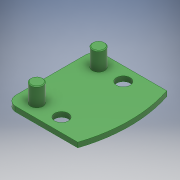
# Autodesk Inventor part: green_part-july21
Saved by Autodesk Inventor 2017 SP1 (Build 210196100, 196)
## iProperties
Created: 2016-07-25
Part Number: green_part-july21
Material: Plastique ABS
Document SubType Name: Modeling
Designer: tmonglon
Density: 1.06 g/cm^3
Appearance: Lisse - Vert forêt foncé
Author: tmonglon
Autodesk Inventor part; units mm, degrees
ref_plane "YZ Plane" through (0, 0, 0) normal (1, 0, 0) x (0, 1, 0)
ref_plane "XZ Plane" through (0, 0, 0) normal (0, 1, 0) x (-1, 0, 0)
ref_plane "XY Plane" through (0, 0, 0) normal (0, 0, 1) x (1, 0, 0)
sketch "Esquisse1" plane through (0, 0, 0) normal (0, 0, 1) x (1, 0, 0)
  line L0 (0, 0) -> (-29, 0)
  line L1 (-29, 0) -> (-29, 36)
  line L2 (-29, 36) -> (0, 36)
  line L3 (-24.5656, 33) -> (-19.5656, 33)
  line L4 (-19.5656, 33) -> (-19.5656, 28)
  line L5 (-19.5656, 28) -> (-24.5656, 28)
  line L6 (-24.5656, 28) -> (-24.5656, 33)
  line L7 (-14.5656, 33) -> (-9.5656, 33)
  line L8 (-9.5656, 33) -> (-9.5656, 28)
  line L9 (-9.5656, 28) -> (-14.5656, 28)
  line L10 (-14.5656, 28) -> (-14.5656, 33)
  line L11 (-24.5656, 8) -> (-19.5656, 8)
  line L12 (-19.5656, 8) -> (-19.5656, 3)
  line L13 (-19.5656, 3) -> (-24.5656, 3)
  line L14 (-24.5656, 3) -> (-24.5656, 8)
  line L15 (-14.5656, 8) -> (-9.5656, 8)
  line L16 (-9.5656, 8) -> (-9.5656, 3)
  line L17 (-9.5656, 3) -> (-14.5656, 3)
  line L18 (-14.5656, 3) -> (-14.5656, 8)
  arc A0 (0, 0) -> (0, 36) centre (-54.0833, 18) ccw
  line L19 (-9.3156, 33.25) -> (-14.8156, 33.25)
  line L20 (-14.8156, 33.25) -> (-14.8156, 27.75)
  line L21 (-14.8156, 27.75) -> (-9.3156, 27.75)
  line L22 (-9.3156, 27.75) -> (-9.3156, 33.25)
  line L23 (-9.3156, 8.25) -> (-14.8156, 8.25)
  line L24 (-14.8156, 8.25) -> (-14.8156, 2.75)
  line L25 (-14.8156, 2.75) -> (-9.3156, 2.75)
  line L26 (-9.3156, 2.75) -> (-9.3156, 8.25)
  dimension "d0" = 36
  dimension "d1" = 29
  dimension "d2" = 5
  dimension "d3" = 5
  dimension "d4" = 5
  dimension "d5" = 5
  dimension "d6" = 20
  dimension "d7" = 5
  dimension "d8" = 3
  dimension "d9" = 57
  dimension "d21" = 5.5
  dimension "d22" = 5.5
  constraints: 54 end point, 13 parallel, 8 point on line, 7 perpendicular, 5 horizontal, 2 point on circle, 1 centre point, 6 other
  measures "d0" distance of L0.end L1.end
  measures "d1" distance of L1.end L2.end
  measures "d2" distance of L5.end L3.start
  measures "d3" distance of L3.start L3.end
  measures "d4" distance of L7.start L7.end
  measures "d5" distance between parallel lines of L10 L4
  measures "d6" distance between parallel lines of L15 L9
  measures "d7" distance of L15.end L16.end
  measures "d8" distance between parallel lines of L0 L17
  measures "d9" radius of A0
  measures "d21" distance of L23.start L23.end
  measures "d22" distance of L20.end L21.end
extrude "Extrusion1" add sketch "Esquisse1" along normal blind 2 contours L0 L1 L2 A0 | L22 L21 L20 L19 | L26 L25 L24 L23
extrude "Extrusion3" add sketch "Esquisse1" along normal blind 9.5 contours L3 L4 L5 L6 | L11 L12 L13 L14
fillet "Congé1" radius 4 2 edges at (-29, 0, 1) (-29, 36, 1)
sketch "Esquisse2" plane through (0, 0, 2) normal (0, 0, 1) x (1, 0, 0)
  line L0 (-9.5656, 8) -> (-9.5656, 3) projected
  line L1 (-9.5656, 3) -> (-14.5656, 3) projected
  line L2 (-14.5656, 3) -> (-14.5656, 8) projected
  line L3 (-14.5656, 8) -> (-9.5656, 8) projected
  line L4 (-19.5656, 8) -> (-19.5656, 3) projected
  line L5 (-19.5656, 3) -> (-24.5656, 3) projected
  line L6 (-24.5656, 3) -> (-24.5656, 8) projected
  line L7 (-24.5656, 8) -> (-19.5656, 8) projected
  line L8 (-9.5656, 33) -> (-9.5656, 28) projected
  line L9 (-9.5656, 28) -> (-14.5656, 28) projected
  line L10 (-14.5656, 28) -> (-14.5656, 33) projected
  line L11 (-14.5656, 33) -> (-9.5656, 33) projected
  line L12 (-19.5656, 33) -> (-19.5656, 28) projected
  line L13 (-19.5656, 28) -> (-24.5656, 28) projected
  line L14 (-24.5656, 28) -> (-24.5656, 33) projected
  line L15 (-24.5656, 33) -> (-19.5656, 33) projected
  arc A0 (-25, 36) -> (-29, 32) centre (-25, 32) ccw projected
  line L16 (-29, 32) -> (-29, 4) projected
  arc A1 (-29, 4) -> (-25, 0) centre (-25, 4) ccw projected
  line L17 (-25, 0) -> (0, 0) projected
  arc A2 (0, 0) -> (0, 36) centre (-54.0833, 18) ccw projected
  line L18 (0, 36) -> (-25, 36) projected
  circle A3 centre (-12.0656, 30.5) radius 2.5
  circle A4 centre (-12.0656, 5.5) radius 2.5
  constraints: 6 tangent, 2 centre point
extrude "Extrusion4" add sketch "Esquisse2" against normal up to surface (2 mm away) contours L0 A4 L3 | L0 L1 A4 | A4 L2 L3 | L1 L2 A4 | L8 A3 L11 | L8 L9 A3 | A3 L10 L11 | L9 L10 A3
sketch "Esquisse3" plane through (0, 0, 9.5) normal (0, 0, 1) x (1, 0, 0)
  circle A0 centre (-12.0656, 5.5) radius 2.5 projected
  line L0 (-19.5656, 8) -> (-19.5656, 3) projected
  line L1 (-19.5656, 3) -> (-24.5656, 3) projected
  line L2 (-24.5656, 3) -> (-24.5656, 8) projected
  line L3 (-24.5656, 8) -> (-19.5656, 8) projected
  circle A1 centre (-12.0656, 30.5) radius 2.5 projected
  line L4 (-19.5656, 33) -> (-19.5656, 28) projected
  line L5 (-19.5656, 28) -> (-24.5656, 28) projected
  line L6 (-24.5656, 28) -> (-24.5656, 33) projected
  line L7 (-24.5656, 33) -> (-19.5656, 33) projected
  arc A2 (-25, 36) -> (-29, 32) centre (-25, 32) ccw projected
  line L8 (-29, 32) -> (-29, 4) projected
  arc A3 (-29, 4) -> (-25, 0) centre (-25, 4) ccw projected
  line L9 (-25, 0) -> (0, 0) projected
  arc A4 (0, 0) -> (0, 36) centre (-54.0833, 18) ccw projected
  line L10 (0, 36) -> (-25, 36) projected
  circle A5 centre (-22.0656, 30.5) radius 2.5
  circle A6 centre (-22.0656, 5.5) radius 2.5
  constraints: 6 tangent, 2 centre point
extrude "Extrusion5" cut sketch "Esquisse3" against normal up to surface (7.5 mm away) contours L0 A6 L3 | L0 L1 A6 | A6 L2 L3 | L1 L2 A6 | L4 A5 L7 | L4 L5 A5 | A5 L6 L7 | L5 L6 A5
sketch "Esquisse4" plane through (0, 0, 2) normal (0, 0, 1) x (1, 0, 0)
  circle A0 centre (-12.0656, 5.5) radius 2.5 projected
  circle A1 centre (-22.0656, 5.5) radius 2.5 projected
  circle A2 centre (-12.0656, 30.5) radius 2.5 projected
  circle A3 centre (-22.0656, 30.5) radius 2.5 projected
  arc A4 (-25, 36) -> (-29, 32) centre (-25, 32) ccw projected
  line L0 (-29, 32) -> (-29, 4) projected
  arc A5 (-29, 4) -> (-25, 0) centre (-25, 4) ccw projected
  line L1 (-25, 0) -> (0, 0) projected
  arc A6 (0, 0) -> (0, 36) centre (-54.0833, 18) ccw projected
  line L2 (0, 36) -> (-25, 36) projected
  circle A7 centre (-12.0656, 30.5) radius 2.75
  circle A8 centre (-12.0656, 5.5) radius 2.75
  dimension "d23" = 5.5
  dimension "d24" = 5.5
  constraints: 2 centre point, 2 coincident
  measures "d23" diameter of A7
  measures "d24" diameter of A8
extrude "Extrusion6" cut sketch "Esquisse4" against normal through all contours A7 | A8
chamfer "Chanfrein1" distance 0.3 angle 45 2 edges at (-24.5656, 5.5, 9.5) (-24.5656, 30.5, 9.5)
